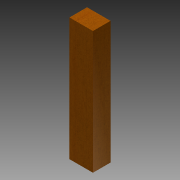
# Autodesk Inventor part: Bottom_Wheel_Supp
Saved by Autodesk Inventor 2014 SP1 (Build 180222100, 222)
## iProperties
Created: 2014-02-22
Part Number: Bottom_Wheel_Supp
Material: Wood
Document SubType Name: Modeling
Designer: tuleu
Density: 0.570257 g/cm^3
Appearance: Yellow Pine - Solid Natural Low Gloss
Author: tuleu
Autodesk Inventor part; units mm, degrees
ref_plane "YZ Plane" through (0, 0, 0) normal (1, 0, 0) x (0, 1, 0)
ref_plane "XZ Plane" through (0, 0, 0) normal (0, 1, 0) x (-1, 0, 0)
sketch "Sketch1" plane through (0, 0, 0) normal (0, 0, 1) x (1, 0, 0)
  line L0 (30, 216.5) -> (-50, 216.5)
  line L1 (-50, 216.5) -> (-50, 276.5)
  line L2 (-50, 276.5) -> (30, 276.5)
  line L3 (30, 276.5) -> (30, 216.5)
  point P0 (0, 0)
  dimension "d0" = 60
  dimension "d1" = 80
  constraints: 8 end point, 2 parallel, 1 horizontal, 1 perpendicular, 1 other
  measures "d0" distance of L2.end L0.start
  measures "d1" distance of L1.end L2.end
ref_plane "Work Plane1" through (-30, -216.5, -268) normal (0, 0, -1) x (0, 1, 0)
extrude "Extrusion1" add sketch "Sketch1" against normal up to surface (268 mm away)
sketch "Sketch2" plane through (0, 0, 0) normal (0, 0, 1) x (1, 0, 0)
  line L0 (30, 216.5) -> (-50, 216.5) projected
  line L1 (30, 276.5) -> (30, 216.5) projected
  line L2 (-50, 276.5) -> (30, 276.5) projected
  line L3 (-50, 216.5) -> (-50, 276.5) projected
  line L4 (30, 216.5) -> (-50, 216.5) projected
  line L5 (30, 276.5) -> (30, 216.5) projected
  line L6 (-50, 276.5) -> (30, 276.5) projected
  line L7 (-50, 216.5) -> (-50, 276.5) projected
  point P0 (0, 0)
extrude "Extrusion2" add sketch "Sketch2" along normal blind 75
sketch "Sketch3" plane through (30, 216.5, -268) normal (0, 0, -1) x (-1, 0, 0)
  line L0 (0, 0) -> (0, 60) projected
  line L1 (80, 0) -> (0, 0) projected
  line L2 (80, 60) -> (80, 0) projected
  line L3 (0, 60) -> (80, 60) projected
  line L4 (0, 0) -> (0, 60) projected
  line L5 (80, 0) -> (0, 0) projected
  line L6 (80, 60) -> (80, 0) projected
  line L7 (0, 60) -> (80, 60) projected
  point P0 (30, -216.5)
extrude "Extrusion3" add sketch "Sketch3" along normal blind 75
body "Solid1"
